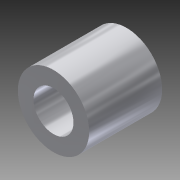
# Autodesk Inventor part: Spacer_ServoTilitBracketArm
Saved by Autodesk Inventor 2015 (Build 190159000, 159)
## iProperties
Created: 2014-05-23
Part Number: Spacer_ServoTilitBracketArm
Material: Generic
Document SubType Name: Modeling
Designer: seaha_000
Density: 1 g/cm^3
Appearance: Default
Mass: 0.141348 g
Surface Area: 2.45834 cm^2
Volume: 0.141348 cm^3
Author: seaha_000
Autodesk Inventor part; units mm, degrees
ref_plane "YZ Plane" through (0, 0, 0) normal (1, 0, 0) x (0, 1, 0)
ref_plane "XZ Plane" through (0, 0, 0) normal (0, 1, 0) x (-1, 0, 0)
ref_plane "XY Plane" through (0, 0, 0) normal (0, 0, 1) x (1, 0, 0)
sketch "Sketch1" plane through (0, 0, 0) normal (0, 0, 1) x (1, 0, 0)
  circle A0 centre (0, 0) radius 1.778
  circle A1 centre (0, 0) radius 3.175
  dimension "d0" = 3.556
  dimension "d1" = 6.35
  constraints: 2 centre point, 2 coincident
  measures "d0" diameter of A0
  measures "d1" diameter of A1
extrude "Extrusion1" add sketch "Sketch1" along normal blind 6.5024
body "Solid1"
